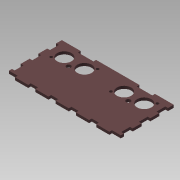
# Autodesk Inventor part: srfbelakang
Saved by Autodesk Inventor 2015 SP1 (Build 190203100, 203)
## iProperties
Created: 2015-02-14
Part Number: srfbelakang
Material: Generic
Document SubType Name: Modeling
Designer: Rafi Kurnia Putra
Density: 1 g/cm^3
Appearance: Default(1)
Author: Rafi Kurnia Putra
Autodesk Inventor part; units mm, degrees
ref_plane "YZ Plane" through (0, 0, 0) normal (1, 0, 0) x (0, 1, 0)
ref_plane "XZ Plane" through (0, 0, 0) normal (0, 1, 0) x (-1, 0, 0)
ref_plane "XY Plane" through (0, 0, 0) normal (0, 0, 1) x (1, 0, 0)
sketch "Sketch1" plane through (0, 0, 0) normal (0, 0, 1) x (1, 0, 0)
  line L0 (-42.0848, 28.5) -> (-42.0848, 31.5)
  line L1 (-24.5848, 28.5) -> (-42.0848, 28.5)
  line L2 (-24.5848, 31.5) -> (-24.5848, 28.5)
  line L3 (-24.5848, 31.5) -> (24.5848, 31.5)
  line L4 (24.5848, 28.5) -> (24.5848, 31.5)
  line L5 (42.0848, 28.5) -> (24.5848, 28.5)
  line L6 (42.0848, 31.5) -> (42.0848, 28.5)
  circle A0 centre (-45.2648, 16.1838) radius 8.115
  circle A1 centre (-22.4048, 16.1838) radius 8.115
  circle A2 centre (-14.7848, 23.4228) radius 1.5875
  circle A3 centre (-52.8848, 8.9448) radius 1.5875
  circle A4 centre (-33.8348, 9.5798) radius 2.5
  circle A5 centre (14.7848, 8.9448) radius 1.5875
  circle A6 centre (22.4048, 16.1838) radius 8.115
  circle A7 centre (33.8348, 9.5798) radius 2.5
  circle A8 centre (45.2648, 16.1838) radius 8.115
  circle A9 centre (52.8848, 23.4228) radius 1.5875
  line L7 (-60.406, 31.5) -> (60.406, -31.5) construction
  line L8 (60.406, 31.5) -> (-60.406, -31.5) construction
  line L9 (-7.5, -31.5) -> (7.5, -31.5)
  line L10 (7.5, -31.5) -> (7.5, -28.5)
  line L11 (-7.5, -28.5) -> (-7.5, -31.5)
  line L12 (-7.5, -31.5) -> (7.5, -28.5) construction
  line L13 (7.5, -31.5) -> (-7.5, -28.5) construction
  line L14 (0, 0) -> (13.8, 0) construction
  line L15 (13.8, 0) -> (13.8, 4) construction
  line L16 (-30.5, -31.5) -> (-15.5, -31.5)
  line L17 (-53.5, -31.5) -> (-38.5, -31.5)
  line L18 (15.5, -31.5) -> (30.5, -31.5)
  line L19 (-7.5, -31.5) -> (7.5, -31.5)
  line L20 (-30.5, -31.5) -> (-15.5, -31.5)
  line L21 (38.5, -31.5) -> (53.5, -31.5)
  line L22 (15.5, -31.5) -> (30.5, -31.5)
  line L23 (-7.5, -31.5) -> (7.5, -31.5)
  line L24 (-15.5, -31.5) -> (-15.5, -28.5)
  line L25 (-15.5, -28.5) -> (-7.5, -28.5)
  line L26 (-30.5, -31.5) -> (-30.5, -28.5)
  line L27 (-30.5, -28.5) -> (-38.5, -28.5)
  line L28 (-38.5, -28.5) -> (-38.5, -31.5)
  line L29 (-53.5, -31.5) -> (-53.5, -28.5)
  line L30 (15.5, -31.5) -> (15.5, -28.5)
  line L31 (15.5, -28.5) -> (7.5, -28.5)
  line L32 (30.5, -31.5) -> (30.5, -28.5)
  line L33 (30.5, -28.5) -> (38.5, -28.5)
  line L34 (38.5, -31.5) -> (38.5, -28.5)
  line L35 (53.5, -31.5) -> (53.5, -28.5)
  line L36 (-60.4057, -31.5) -> (-60.4057, -31.4998)
  line L37 (-63.4057, 5) -> (-63.4057, 15)
  line L38 (-63.4057, -5) -> (-63.4057, -15)
  line L39 (-63.4057, -25) -> (-63.4057, -28.5)
  line L40 (-63.4057, 25) -> (-63.4057, 31.5)
  line L41 (-42.0848, 31.5) -> (-63.4057, 31.5)
  line L42 (-63.4057, 25) -> (-60.4057, 25)
  line L43 (-60.4057, 25) -> (-60.4057, 15)
  line L44 (-63.4057, 15) -> (-60.4057, 15)
  line L45 (-63.4057, 5) -> (-60.4057, 5)
  line L46 (-60.4057, 5) -> (-60.4057, -5)
  line L47 (-60.4057, -5) -> (-63.4057, -5)
  line L48 (-63.4057, -15) -> (-60.4057, -15)
  line L49 (-60.4057, -15) -> (-60.4057, -25)
  line L50 (-60.4057, -25) -> (-63.4057, -25)
  line L51 (-63.4057, -28.5) -> (-53.5, -28.5)
  line L52 (0, 0) -> (0, 18) construction
  line L53 (60.4057, -31.5) -> (60.4057, -31.4998)
  line L54 (63.4057, 5) -> (63.4057, 15)
  line L55 (63.4057, -5) -> (63.4057, -15)
  line L56 (63.4057, -25) -> (63.4057, -28.5)
  line L57 (63.4057, 25) -> (63.4057, 31.5)
  line L58 (42.0848, 31.5) -> (63.4057, 31.5)
  line L59 (63.4057, 25) -> (60.4057, 25)
  line L60 (60.4057, 25) -> (60.4057, 15)
  line L61 (63.4057, 15) -> (60.4057, 15)
  line L62 (63.4057, 5) -> (60.4057, 5)
  line L63 (60.4057, 5) -> (60.4057, -5)
  line L64 (60.4057, -5) -> (63.4057, -5)
  line L65 (63.4057, -15) -> (60.4057, -15)
  line L66 (60.4057, -15) -> (60.4057, -25)
  line L67 (60.4057, -25) -> (63.4057, -25)
  line L68 (63.4057, -28.5) -> (53.5, -28.5)
  point P0 (0, 0)
  point P1 (0, -30)
  dimension "d0" = 15
  dimension "d1" = 3
  dimension "d5" = 23
  dimension "d8" = 23
  dimension "d11" = 3
  dimension "d12" = 3
  dimension "d13" = 90
  dimension "d14" = 3
  dimension "d17" = 3
  dimension "d18" = 10
  dimension "d20" = 10
  constraints: 138 end point, 16 symmetric about line, 11 vertical, 10 centre point, 9 perpendicular, 7 horizontal, 6 point on line, 3 midpoint, 2 parallel, 24 other
  measures "d0" distance of L11.start L10.end
  measures "d1" distance of L10.end L9.end
  measures "d5" distance of L9.start L16.start
  measures "d8" distance of L9.start L18.start
  measures "d11" distance of L22.start L30.end
  measures "d12" distance of L22.end L32.end
  measures "d13" angle of L32 L33
  measures "d14" distance of L21.end L35.end
  measures "d17" distance of L37.end L43.end
  measures "d18" distance of L37.start L37.end
  measures "d20" distance of L38.start L38.end
extrude "Extrusion1" add sketch "Sketch1" along normal mid plane 3
body "Solid1"
